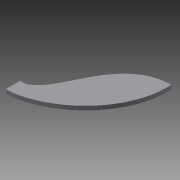
# Autodesk Inventor part: cola
Saved by Autodesk Inventor 2015 (Build 190159000, 159)
## iProperties
Created: 2017-11-29
Part Number: cola
Material: Generic
Document SubType Name: Modeling
Designer: Max
Density: 1 g/cm^3
Appearance: Default
Author: Max
Autodesk Inventor part; units mm, degrees
ref_plane "YZ Plane" through (0, 0, 0) normal (1, 0, 0) x (0, 1, 0)
ref_plane "XZ Plane" through (0, 0, 0) normal (0, 1, 0) x (-1, 0, 0)
ref_plane "XY Plane" through (0, 0, 0) normal (0, 0, 1) x (1, 0, 0)
sketch "Sketch1" plane through (0, 0, 0) normal (0, 0, 1) x (1, 0, 0)
  line L0 (0, 0) -> (8, 0)
  line L1 (8, 20) -> (0, 20)
  line L2 (0, 20) -> (0, 0)
  line L3 (8, 0) -> (68.3243, 10) construction
  line L4 (68.3243, 10) -> (114.2453, 65.2975) construction
  line L5 (114.2453, 65.2975) -> (110.2522, 120.7022) construction
  spline S0 degree 3 poles (8, 0) (68.3243, 10) (114.2453, 65.2975) (110.2522, 120.7022) knots 1 1 1 1 2 2 2 2
  line L6 (8, 20) -> (38.1621, 35.0478) construction
  line L7 (38.1621, 35.0478) -> (38.1621, 87.6603) construction
  line L8 (38.1621, 87.6603) -> (68.3243, 120.7022) construction
  line L9 (68.3243, 120.7022) -> (110.2522, 120.7022) construction
  spline S1 degree 4 poles (8, 20) (38.1621, 35.0478) (38.1621, 87.6603) (68.3243, 120.7022) (110.2522, 120.7022) knots 1 1 1 1 1 2 2 2 2 2
  constraints: 6 end point, 2 horizontal, 1 parallel, 1 vertical, 6 other
extrude "Extrusion1" add sketch "Sketch1" along normal blind 5.5
body "Solid1"
